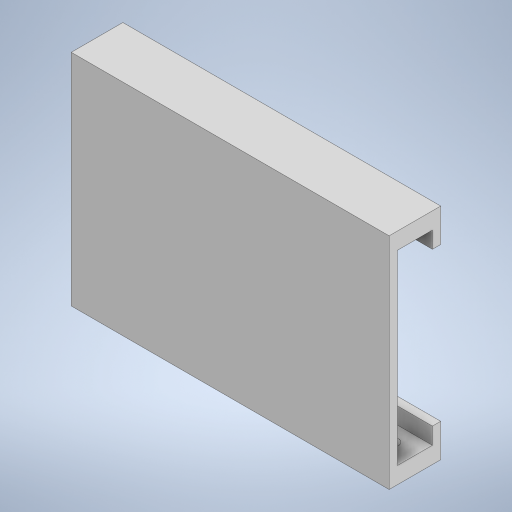
# Autodesk Inventor part: CaseV1
Saved by Autodesk Inventor 2024 (Build 280153000, 153)
## iProperties
Created: 2024-01-03
Part Number: CaseV1
Material: Generisch
Document SubType Name: Modeling
Designer: chris
Density: 1 g/cm^3
Appearance: Vorgabe
Author: chris
Autodesk Inventor part; units mm, degrees
ref_plane "YZ Plane" through (0, 0, 0) normal (1, 0, 0) x (0, 1, 0)
ref_plane "XZ Plane" through (0, 0, 0) normal (0, 1, 0) x (-1, 0, 0)
ref_plane "XY Plane" through (0, 0, 0) normal (0, 0, 1) x (1, 0, 0)
sketch "Skizze1" plane through (0, 0, 0) normal (0, 1, 0) x (-1, 0, 0)
  line L0 (-18.1, -11.2) -> (18.1, -11.2)
  line L1 (18.1, -11.2) -> (18.1, 11.2)
  line L2 (18.1, 11.2) -> (-18.1, 11.2)
  line L3 (-18.1, 11.2) -> (-18.1, -11.2)
  line L4 (-18.1, -11.2) -> (18.1, 11.2) construction
  line L5 (18.1, -11.2) -> (-18.1, 11.2) construction
  point P0 (0, 0)
  dimension "d0" = 36.2
  dimension "d1" = 22.4
  constraints: 12 end point, 2 midpoint, 2 parallel, 1 horizontal, 1 perpendicular
  measures "d0" distance between parallel lines of L3 L1
  measures "d1" distance between parallel lines of L0 L2
extrude "Extrusion1" add sketch "Skizze1" along normal blind 1
sketch "Skizze2" plane through (0, 0, 0) normal (0, 1, 0) x (-1, 0, 0)
  line L0 (18.1, -11.2) -> (18.1, 11.2) projected
  line L1 (-18.1, -11.2) -> (18.1, -11.2)
  line L2 (18.1, -11.2) -> (18.1, 11.2)
  line L3 (18.1, 11.2) -> (-18.1, 11.2)
  line L4 (-18.1, 11.2) -> (-18.1, -11.2)
  line L5 (-18.1, -11.2) -> (18.1, 11.2) construction
  line L6 (18.1, -11.2) -> (-18.1, 11.2) construction
  line L7 (-20.1, -13.2) -> (20.1, -13.2)
  line L8 (20.1, -13.2) -> (20.1, 13.2)
  line L9 (20.1, 13.2) -> (-20.1, 13.2)
  line L10 (-20.1, 13.2) -> (-20.1, -13.2)
  line L11 (-20.1, -13.2) -> (20.1, 13.2) construction
  line L12 (20.1, -13.2) -> (-20.1, 13.2) construction
  line L13 (-18.1, -11.2) -> (-18.1, -13.2)
  line L14 (-18.1, 11.2) -> (-18.1, 13.2)
  point P0 (0, 0)
  dimension "d4" = 2
  dimension "d5" = 2
  constraints: 28 end point, 4 midpoint, 4 parallel, 4 perpendicular, 2 horizontal, 2 point on line
  measures "d4" distance between parallel lines of L8 L0
  measures "d5" distance between parallel lines of L7 L1
extrude "Extrusion2" add sketch "Skizze2" along normal blind 5.2 contours L0 L3 L14 L9 L8 L7 L13 L1
sketch "Skizze3" plane through (0, 5.2, 0) normal (0, 1, 0) x (1, 0, 0)
  line L0 (18.1, -13.2) -> (18.1, 13.2) projected
  line L1 (-16.1, -9.2) -> (18.1, -9.2)
  line L2 (18.1, -9.2) -> (18.1, 9.2)
  line L3 (18.1, 9.2) -> (-16.1, 9.2)
  line L4 (-16.1, 9.2) -> (-16.1, -9.2)
  line L5 (-18.1, 11.2) -> (18.1, 11.2) projected
  line L6 (-18.1, -11.2) -> (-18.1, 11.2) projected
  line L7 (18.1, -11.2) -> (-18.1, -11.2) projected
  line L8 (-20.1, -13.2) -> (18.1, -13.2) projected
  line L9 (-20.1, -13.2) -> (18.1, -13.2)
  line L10 (18.1, -13.2) -> (18.1, 13.2)
  line L11 (18.1, 13.2) -> (-20.1, 13.2)
  line L12 (-20.1, 13.2) -> (-20.1, -13.2)
  point P0 (0, 0)
  dimension "d8" = 2
  dimension "d9" = 2
  dimension "d10" = 2
  constraints: 16 end point, 4 parallel, 2 horizontal, 2 perpendicular, 1 point on line
  measures "d8" distance between parallel lines of L5 L3
  measures "d9" distance between parallel lines of L6 L4
  measures "d10" distance between parallel lines of L7 L1
extrude "Extrusion3" add sketch "Skizze3" along normal blind 1 contours L8 L12 L11 L0 L5 L6 L7 | L7 L6 L5 L0 L3 L4 L1
sketch "Skizze4" plane through (18.1, 1, 11.2) normal (0, 0, -1) x (-1, 0, 0)
  line L0 (0, 4.2) -> (34.2, 4.2) construction
  line L1 (2.75, 4.2) -> (2.75, 0) construction
  line L2 (0, 0) -> (36.2, 0) construction
  circle A0 centre (2.75, 2.1) radius 0.75
  line L3 (0, -1) -> (0, 5.2) projected
  point P0 (18.1, -1)
  dimension "d13" = 1.5
  dimension "d14" = 2
  constraints: 2 end point, 2 point on line, 1 centre point, 1 midpoint, 1 vertical
  measures "d13" diameter of A0
  measures "d14" distance edge to line of A0 L3
extrude "Extrusion4" add sketch "Skizze4" along normal blind 0.3 draft -50
mirror "Spiegeln1" about plane through (0, 0, 0) normal (0, 0, 1) of "Extrusion4"
